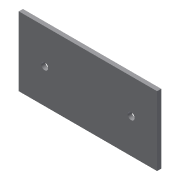
# Autodesk Inventor part: Nano Mounting Plate
Saved by Autodesk Inventor 2015 (Build 190159000, 159)
## iProperties
Created: 2015-02-15
Part Number: Nano Mounting Plate
Material: Generic
Document SubType Name: Sheet Metal
Designer: Noah
Density: 1 g/cm^3
Sheet Metal Rule: Default
Appearance: Default
Author: Noah
Autodesk Inventor part; units mm, degrees
ref_plane "YZ Plane" through (0, 0, 0) normal (1, 0, 0) x (0, 1, 0)
ref_plane "XZ Plane" through (0, 0, 0) normal (0, 1, 0) x (-1, 0, 0)
ref_plane "XY Plane" through (0, 0, 0) normal (0, 0, 1) x (1, 0, 0)
sketch "Sketch1" plane through (0, 0, 0) normal (0, 0, 1) x (1, 0, 0)
  line L0 (0, 0) -> (-101.6, 0)
  line L1 (-101.6, 0) -> (-101.6, 50.8)
  line L2 (-101.6, 50.8) -> (0, 50.8)
  line L3 (0, 50.8) -> (0, 0)
  circle A0 centre (-82.55, 25.4) radius 2.5527
  circle A1 centre (-19.05, 25.4) radius 2.5527
  dimension "holewidth" = 5.1054
  dimension "d1" = 5.1054
  dimension "d2" = 50.8
  dimension "d3" = 101.6
  dimension "d6" = 63.5
  dimension "d7" = 19.05
  dimension "d8" = 25.4
  dimension "d9" = 19.05
  measures "holewidth" diameter of A0
  measures "d1" diameter of A1
  measures "d2" distance of L2.end L0.start
  measures "d3" distance of L1.end L2.end
  measures "d6" distance of A1.centre A0.centre
  measures "d7" distance from line of L1 A0.centre
  measures "d8" distance from line of L0 A0.centre
  measures "d9" distance from line of A1.centre L3
extrude "Plate1" add sketch "Sketch1" along normal blind 3.048
equation "\"d1\" = holewidth"
equation "\"BendRadius\" = Thickness"
equation "\"BendReliefWidth\" = Thickness"
equation "\"BendReliefDepth\" = 0.5 * Thickness"
equation "\"CornerReliefSize\" = 4 * Thickness"
equation "\"MinimumRemnant\" = 2 * Thickness"
equation "\"TransitionRadius\" = BendRadius"
equation "\"JacobiRadiusSize\" = BendRadius"
equation "\"GapSize\" = Thickness"
equation "\"d10\" = BendRadius"
equation "\"Thickness\" = 3.048"
body "Solid1"
